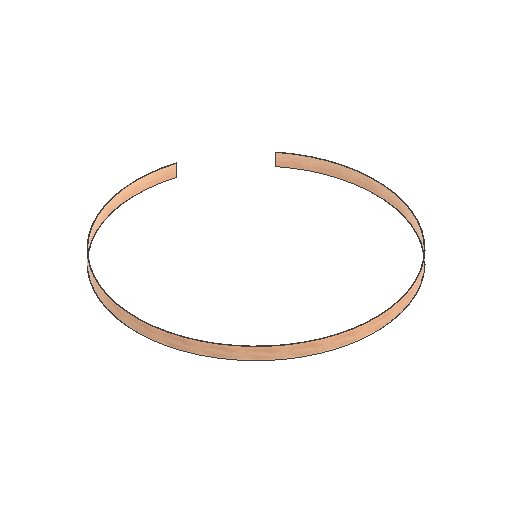
# Autodesk Inventor part: Edge Band - Platform D Inner
Saved by Autodesk Inventor 2021 (Build 250183000, 183)
## iProperties
Created: 2020-05-12
Part Number: Edge Band - Platform D Inner
Material: Wood (Birch)
Document SubType Name: Modeling
Designer: Dan Wikman
Density: 0.55 g/cm^3
Appearance: Birch - Natural Polished
Mass: 1210.24 g
Surface Area: 11450.4 cm^2
Volume: 2200.43 cm^3
Author: Dan Wikman
Autodesk Inventor part; units mm, degrees
ref_plane "YZ Plane" through (0, 0, 0) normal (1, 0, 0) x (0, 1, 0)
ref_plane "XZ Plane" through (0, 0, 0) normal (0, 1, 0) x (-1, 0, 0)
ref_plane "XY Plane" through (0, 0, 0) normal (0, 0, 1) x (1, 0, 0)
sketch "Sketch1" plane through (0, 0, 0) normal (0, 1, 0) x (-1, 0, 0)
  circle A0 centre (0, 0) radius 971.25
  circle A1 centre (0, 0) radius 967.25
  dimension "d0" = 1942.5
  dimension "d1" = 1934.5
  constraints: 2 centre point, 2 coincident
  measures "d0" diameter of A0
  measures "d1" diameter of A1
extrude "Extrusion1" add sketch "Sketch1" along normal blind 100
sketch "Sketch2" plane through (0, 0, 0) normal (0, -1, 0) x (1, 0, 0)
  line L0 (-1202.4006, -424.0965) -> (-929.1876, -282.72) projected
  line L1 (-601.6735, -761.7695) -> (-832.5638, -965.0384) projected
  circle A0 centre (0, 0) radius 967.25 projected
  line L2 (-599.0233, -759.4364) -> (-602.0753, -762.1233)
  circle A1 centre (0, 0) radius 971.25 projected
  line L3 (-925.578, -280.8522) -> (-929.1876, -282.72)
  point P0 (-929.1905, -282.7216)
  constraints: 4 end point, 2 point on circle, 1 collinear, 1 point on line, 2 other
extrude "Extrusion2" cut sketch "Sketch2" against normal blind 100 contours L0 L3 A0 L2 L1 A1 picked at (-908.76, -334.5466)
body "Solid1"
